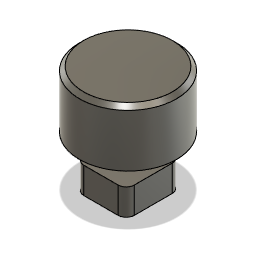
chassis_v1.0_printing (Autodesk Fusion 360 archive; units mm, degrees)
design "encoder"
Autodesk Fusion 360 part; units mm, degrees
sketch "Sketch1" plane through (0, 0, 0) normal (0, 1, 0) x (1, 0, 0)
  line L0 (6.25, -6.7) -> (-6.25, -6.7)
  line L1 (-6.25, -6.7) -> (-6.25, 6.7)
  line L2 (-6.25, 6.7) -> (6.25, 6.7)
  line L3 (6.25, 6.7) -> (6.25, -6.7)
  line L4 (6.25, -6.7) -> (-6.25, 6.7) construction
  line L5 (-6.25, -6.7) -> (6.25, 6.7) construction
  circle A0 centre (0, 0) radius 3
  circle A1 centre (0, 0) radius 3.5
  line L6 (-2.5, -4.3301) -> (2.5, 4.3301) construction
  line L7 (-2.5, 4.3301) -> (2.5, -4.3301) construction
  line L8 (-5, 0) -> (5, 0) construction
  line L9 (-2.5, -4.3301) -> (2.5, -4.3301)
  line L10 (2.5, -4.3301) -> (5, 0)
  line L11 (5, 0) -> (2.5, 4.3301)
  line L12 (2.5, 4.3301) -> (-2.5, 4.3301)
  line L13 (-2.5, 4.3301) -> (-5, 0)
  line L14 (-5, 0) -> (-2.5, -4.3301)
  circle A2 centre (0, 0) radius 12
  dimension "d1" = 13.4
  dimension "d2" = 12.5
  dimension "d3" = 6
  dimension "d4" = 7
  dimension "d16" = 10
  dimension "d17" = 60
  dimension "d18" = 60
  dimension "d23" = 24
  constraint horizontal L0
  constraint perpendicular L0 L1
  constraint parallel L0 L2
  constraint parallel L1 L3
  constraint coincident L4 A0.centre
  constraint coincident L5 A0.centre
  constraint coincident A0.centre A1.centre
  constraint midpoint L6 A0.centre
  constraint midpoint A0.centre L7
  constraint equal L6 L7
  constraint horizontal L8
  constraint midpoint A0.centre L8
  constraint equal L6 L8
  measures "d1" distance of L0.start L2.end
  measures "d2" distance of L1.end L2.end
  measures "d3" diameter of A0
  measures "d4" diameter of A1
  measures "d16" distance of L6.start L6.end
  measures "d17" angle of L6 L8
  measures "d18" angle of L7 L8
  measures "d23" diameter of A2
extrude "Extrude1" add sketch "Sketch1" along normal blind 6.5 contours L0 L1 L2 L3 | A0 | A1 | L9 L10 L11 L12 L13 L14
extrude "Extrude2" add sketch "Sketch1" along normal blind 7 from surface at 6.5 contours A0 | A1
thread "Thread1" "ISO Metric profile 7.0 M7x1 6g" major diameter 6.884 minor diameter 5.744 pitch 1 angle 60 resizes the face on face at (3.4826, 11.1667, 0.3485)
extrude "Extrude3" add sketch "Sketch1" along normal blind 13 from surface at 13.5 contours A0
fillet "Fillet1" radius 2 4 edges at (-6.25, 3.25, 6.7) (6.25, 3.25, 6.7) (-6.25, 3.25, -6.7) (6.25, 3.25, -6.7)
extrude "Extrude5" add sketch "Sketch1" against normal blind 14 from surface at 26.5 contours L0 L1 L2 L3 | A0 | A1 | L9 L10 L11 L12 L13 L14 | A2
chamfer "Chamfer1" distance 1 angle 45 1 edges at (-11.1879, 26.5, -4.3394)
